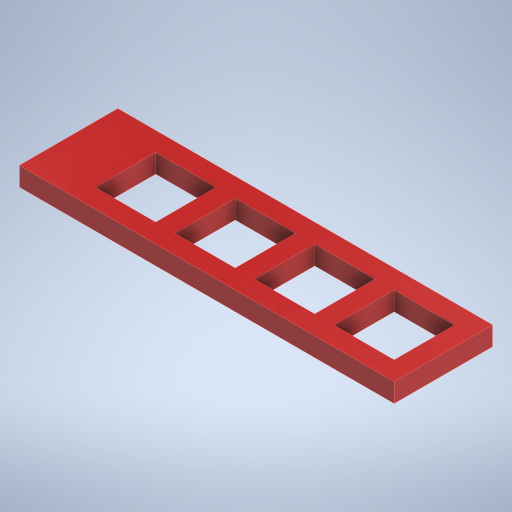
# Autodesk Inventor part: NewSlide
Saved by Autodesk Inventor 2024 (Build 280153000, 153)
## iProperties
Created: 2023-10-24
Part Number: NewSlide
Material: Generic
Document SubType Name: Modeling
Designer: flynf
Density: 1 g/cm^3
Appearance: Red
Author: flynf
Autodesk Inventor part; units mm, degrees
ref_plane "YZ Plane" through (0, 0, 0) normal (1, 0, 0) x (0, 1, 0)
ref_plane "XZ Plane" through (0, 0, 0) normal (0, 1, 0) x (-1, 0, 0)
ref_plane "XY Plane" through (0, 0, 0) normal (0, 0, 1) x (1, 0, 0)
sketch "Sketch1" plane through (0, 0, 0) normal (0, 1, 0) x (-1, 0, 0)
  line L0 (0, 0) -> (-251.46, 0)
  line L1 (-251.46, 0) -> (-251.46, -66.04)
  line L2 (-251.46, -66.04) -> (0, -66.04)
  line L3 (0, -66.04) -> (0, 0)
  dimension "d0" = 251.46
  dimension "d1" = 66.04
  constraints: 8 end point, 2 parallel, 1 horizontal, 1 perpendicular
  measures "d0" distance of L1.end L2.end
  measures "d1" distance of L0.end L1.end
extrude "Extrusion1" add sketch "Sketch1" along normal blind 12.7
sketch "Sketch2" plane through (0, 12.7, 0) normal (0, 1, 0) x (1, 0, 0)
  line L0 (198.12, 12.7) -> (238.76, 12.7)
  line L1 (238.76, 12.7) -> (238.76, 53.34)
  line L2 (238.76, 53.34) -> (198.12, 53.34)
  line L3 (198.12, 53.34) -> (198.12, 12.7)
  line L4 (251.46, 66.04) -> (0, 66.04) projected
  line L5 (0, 0) -> (251.46, 0) projected
  line L6 (251.46, 0) -> (251.46, 66.04) projected
  line L7 (144.78, 12.7) -> (185.42, 12.7)
  line L8 (185.42, 12.7) -> (185.42, 53.34)
  line L9 (185.42, 53.34) -> (144.78, 53.34)
  line L10 (144.78, 53.34) -> (144.78, 12.7)
  line L11 (91.44, 12.7) -> (132.08, 12.7)
  line L12 (132.08, 12.7) -> (132.08, 53.34)
  line L13 (132.08, 53.34) -> (91.44, 53.34)
  line L14 (91.44, 53.34) -> (91.44, 12.7)
  line L15 (78.74, 12.7) -> (38.1, 12.7)
  line L16 (38.1, 12.7) -> (38.1, 53.34)
  line L17 (38.1, 53.34) -> (78.74, 53.34)
  line L18 (78.74, 53.34) -> (78.74, 12.7)
  dimension "d4" = 12.7
  dimension "d5" = 12.7
  dimension "d6" = 12.7
  dimension "d7" = 40.64
  dimension "d8" = 12.7
  dimension "d9" = 12.7
  dimension "d10" = 12.7
  dimension "d11" = 40.64
  dimension "d12" = 12.7
  dimension "d13" = 12.7
  dimension "d14" = 12.7
  dimension "d15" = 40.64
  dimension "d16" = 12.7
  dimension "d17" = 12.7
  dimension "d18" = 12.7
  dimension "d19" = 40.64
  constraints: 32 end point, 8 parallel, 4 horizontal, 4 perpendicular
  measures "d4" distance between parallel lines of L4 L2
  measures "d5" distance between parallel lines of L0 L5
  measures "d6" distance between parallel lines of L6 L1
  measures "d7" distance of L1.end L2.end
  measures "d8" distance between parallel lines of L4 L9
  measures "d9" distance between parallel lines of L5 L7
  measures "d10" distance between parallel lines of L3 L8
  measures "d11" distance of L8.end L9.end
  measures "d12" distance between parallel lines of L4 L13
  measures "d13" distance between parallel lines of L5 L11
  measures "d14" distance between parallel lines of L10 L12
  measures "d15" distance between parallel lines of L12 L14
  measures "d16" distance between parallel lines of L4 L17
  measures "d17" distance between parallel lines of L5 L15
  measures "d18" distance between parallel lines of L18 L14
  measures "d19" distance between parallel lines of L18 L16
extrude "Extrusion2" cut sketch "Sketch2" against normal blind 12.7
body "Solid1"
